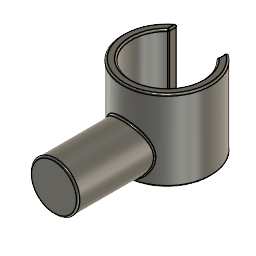
Hands (Autodesk Fusion 360 archive; units mm, degrees)
design "LeftHand"
part number: 2026-05-19-15-14-27-617
Autodesk Fusion 360 part; units mm, degrees
sketch "HandOutline" plane through (0, 0, 0) normal (0, 0, 1) x (1, 0, 0)
  circle A0 centre (0, 0) radius 1.7272
  circle A1 centre (0, 0) radius 1.397
  line L0 (-0.9525, 1.4408) -> (-0.9525, 1.0219)
  line L1 (0.9525, 1.4408) -> (0.9525, 1.0219)
  line L2 (0, 1.7272) -> (0, -1.7272) construction
  dimension "d1" = 3.4544
  dimension "d2" = 2.794
  dimension "d3" = 1.905
  constraint coincident A0.centre A1.centre
  constraint concentric A0 A1
  constraint coincident A0 L0.start
  constraint coincident A1 L0.end
  constraint vertical L0
  constraint coincident A0 L1.start
  constraint coincident A1 L1.end
  constraint parallel L0 L1
  constraint coincident A0 L2.start
  constraint coincident A0 L2.end
  constraint vertical L2
  constraint symmetric L0 L1 L2
  measures "d1" diameter of A0
  measures "d2" diameter of A1
  measures "d3" distance of L0 L1
extrude "Extrude1" add sketch "HandOutline" along normal blind 2.159 and the other way blind 1.016 contours A0 A1 L0 L1 picked at (-1.1455, 1.1363)
sketch "HandJoint" plane through (0, 0, 0) normal (0, 1, 0) x (1, 0, 0)
  circle A0 centre (0, 0) radius 0.9525
  dimension "d8" = 1.905
  constraint coincident A0.centre origin
  measures "d8" diameter of A0
extrude "Extrude2" add sketch "HandJoint" against normal blind 4.445
delete_face "DeleteFace1" 1 faces at (-0.0029, -0.4657, -0.9525)
fillet "Fillet1" radius 0.0635 2 edges at (-0.888, -4.445, -0.3444) (-0.9525, -1.4408, 0) 4 faces at (0, -1.6141, 2.159) (-0.9525, 1.3012, 0.0423) (0.9525, 1.3012, 0.0423) (0, -1.6141, -1.016)
named bodies: "Hand"
